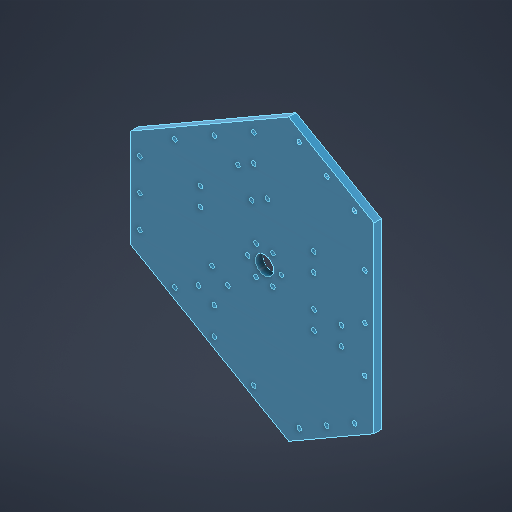
# Autodesk Inventor part: đế trên
Saved by Autodesk Inventor 2027.1 (Build 311270010, 270A)
## iProperties
Created: 2026-08-08
Part Number: đế trên
Material: Generic
Document SubType Name: Sheet Metal
Designer: MSI
Density: 1 g/cm^3
Sheet Metal Rule: Default_mm
Appearance: Sky Blue Dark
Author: MSI
Autodesk Inventor part; units mm, degrees
ref_plane "YZ Plane" through (0, 0, 0) normal (1, 0, 0) x (0, 1, 0)
ref_plane "XZ Plane" through (0, 0, 0) normal (0, 1, 0) x (-1, 0, 0)
ref_plane "XY Plane" through (0, 0, 0) normal (0, 0, 1) x (1, 0, 0)
sketch "Sketch1" plane through (0, 0, 0) normal (0, 0, 1) x (1, 0, 0)
  line L0 (120, 0) -> (120, -100)
  line L1 (120, 0) -> (120, 100)
  line L2 (-60, 103.923) -> (26.6025, 153.923)
  line L3 (-60, 103.923) -> (-146.6025, 53.923)
  line L4 (-60, -103.923) -> (-146.6025, -53.923)
  line L5 (-60, -103.923) -> (26.6025, -153.923)
  line L6 (26.6025, 153.923) -> (120, 100)
  line L7 (120, -100) -> (26.6025, -153.923)
  line L8 (-146.6025, -53.923) -> (-146.6025, 53.923)
  circle A0 centre (0, 0) radius 10
  dimension "d5" = 360
  constraints: 18 end point, 3 vertical, 1 centre point, 1 coincident, 16 other
extrude "Extrusion1" add sketch "Sketch1" along normal blind 8
sketch "Sketch2" plane through (0, 0, 8) normal (0, 0, 1) x (1, 0, 0)
  circle A0 centre (84.2544, -15) radius 2.5
  line L0 (120, -100) -> (120, 100) projected
  circle A1 centre (84.2544, -35) radius 2.5
  circle A2 centre (54.2544, -15) radius 2.5
  circle A3 centre (54.2544, -35) radius 2.5
  circle A4 centre (-14.1368, 54.4857) radius 2.5
  circle A5 centre (-29.1368, 80.4664) radius 2.5
  circle A6 centre (-11.8163, 90.4664) radius 2.5
  circle A7 centre (3.1837, 64.4857) radius 2.5
  circle A8 centre (-40.1176, -39.4857) radius 2.5
  circle A9 centre (-55.1176, -65.4664) radius 2.5
  circle A10 centre (-72.4381, -55.4664) radius 2.5
  circle A11 centre (-57.4381, -29.4857) radius 2.5
  point P0 (0, 0)
  point P1 (120, 0)
  dimension "d11" = 5
  dimension "d12" = 15
  dimension "d13" = 5
  dimension "d14" = 20
  dimension "d15" = 5
  dimension "d16" = 5
  dimension "d17" = 20
  dimension "d18" = 30
  dimension "d21" = 360
  constraints: 12 centre point, 1 midpoint, 25 other
  measures "d11" diameter of A0
  measures "d12" vertical distance of point (120, 0) A0.centre
  measures "d13" diameter of A1
  measures "d14" distance of A1.centre A0.centre
  measures "d15" diameter of A2
  measures "d16" diameter of A3
  measures "d17" distance of A3.centre A2.centre
  measures "d18" distance of A1.centre A3.centre
extrude "Extrusion2" cut sketch "Sketch2" against normal blind 8
sketch "Sketch3" plane through (0, 0, 8) normal (0, 0, 1) x (1, 0, 0)
  circle A0 centre (-136.6025, 35) radius 2.5
  circle A1 centre (-136.6025, 0) radius 2.5
  circle A2 centre (-136.6025, -35) radius 2.5
  line L0 (-146.6025, 53.923) -> (-146.6025, -53.923) projected
  circle A3 centre (37.9904, -135.8013) radius 2.5
  circle A4 centre (68.3013, -118.3013) radius 2.5
  circle A5 centre (98.6122, -100.8013) radius 2.5
  circle A6 centre (98.6122, 100.8013) radius 2.5
  circle A7 centre (68.3013, 118.3013) radius 2.5
  circle A8 centre (37.9904, 135.8013) radius 2.5
  point P0 (0, 0)
  point P1 (-146.6025, 0)
  point P2 (-146.6025, 0)
  dimension "d25" = 5
  dimension "d26" = 5
  dimension "d27" = 5
  dimension "d28" = 35
  dimension "d29" = 35
  dimension "d30" = 0
  dimension "d33" = 360
  dimension "d82" = 10
  dimension "d83" = 10
  constraints: 9 centre point, 2 midpoint, 19 other
  measures "d25" diameter of A0
  measures "d26" diameter of A1
  measures "d27" diameter of A2
  measures "d28" distance of A1.centre A0.centre
  measures "d29" distance of A2.centre A1.centre
  measures "d30" vertical distance of point (-146.603, 0) A1.centre
  measures "d82" distance from line of L0 A0.centre
  measures "d83" distance of point (-146.603, 0) A1.centre
extrude "Extrusion3" cut sketch "Sketch3" against normal blind 8
sketch "Sketch5" plane through (0, 0, 8) normal (0, 0, 1) x (1, 0, 0)
  circle A0 centre (18.3712, 0) radius 2.5
  circle A1 centre (9.1856, 15.9099) radius 2.5
  circle A2 centre (-9.1856, 15.9099) radius 2.5
  circle A3 centre (-18.3712, 0) radius 2.5
  circle A4 centre (-9.1856, -15.9099) radius 2.5
  circle A5 centre (9.1856, -15.9099) radius 2.5
  point P0 (0, 0)
  dimension "d51" = 5
  dimension "d54" = 360
  constraints: 6 centre point, 13 other
  measures "d51" diameter of A0
extrude "Extrusion5" cut sketch "Sketch5" against normal blind 8
sketch "Sketch6" plane through (0, 0, 8) normal (0, 0, 1) x (1, 0, 0)
  circle A0 centre (53.9473, 40) radius 2.5
  circle A1 centre (53.9473, 20) radius 2.5
  line L0 (120, -100) -> (120, 100) projected
  circle A2 centre (-70.3891, 40) radius 2.5
  circle A3 centre (-70.3891, 20) radius 2.5
  point P0 (0, 0)
  point P1 (120, 0)
  dimension "d58" = 5
  dimension "d59" = 5
  dimension "d60" = 20
  dimension "d61" = 20
  dimension "d62" = 5
  dimension "d63" = 5
  dimension "d64" = 20
  constraints: 4 centre point, 1 midpoint
  measures "d58" diameter of A0
  measures "d59" diameter of A1
  measures "d60" vertical distance of point (120, 0) A1.centre
  measures "d61" distance of A1.centre A0.centre
  measures "d62" diameter of A2
  measures "d63" diameter of A3
  measures "d64" distance of A3.centre A2.centre
extrude "Extrusion6" cut sketch "Sketch6" against normal blind 8
sketch "Sketch7" plane through (0, 0, 8) normal (0, 0, 1) x (1, 0, 0)
  circle A0 centre (110, 0) radius 2.5
  circle A1 centre (110, 50) radius 2.5
  circle A2 centre (110, -50) radius 2.5
  line L0 (120, -100) -> (120, 100) projected
  circle A3 centre (-98.3013, 70.2628) radius 2.5
  circle A4 centre (-55, 95.2628) radius 2.5
  circle A5 centre (-11.6987, 120.2628) radius 2.5
  circle A6 centre (-11.6987, -120.2628) radius 2.5
  circle A7 centre (-55, -95.2628) radius 2.5
  circle A8 centre (-98.3013, -70.2628) radius 2.5
  point P0 (0, 0)
  point P1 (120, 0)
  point P2 (120, 0)
  point P3 (120, 0)
  dimension "d68" = 5
  dimension "d69" = 5
  dimension "d70" = 5
  dimension "d71" = 50
  dimension "d72" = 50
  dimension "d75" = 360
  dimension "d77" = 10
  dimension "d78" = 10
  dimension "d79" = 10
  constraints: 9 centre point, 3 midpoint, 19 other
  measures "d68" diameter of A0
  measures "d69" diameter of A1
  measures "d70" diameter of A2
  measures "d71" vertical distance of point (120, 0) A1.centre
  measures "d72" vertical distance of point (120, 0) A2.centre
  measures "d77" distance of point (120, 0) A0.centre
  measures "d78" distance from line of L0 A1.centre
  measures "d79" distance from line of L0 A2.centre
extrude "Extrusion7" cut sketch "Sketch7" against normal blind 8
equation "\"BendRadius\" = Thickness"
equation "\"BendReliefWidth\" = Thickness"
equation "\"BendReliefDepth\" = 0.5 * Thickness"
equation "\"CornerReliefSize\" = 4 * Thickness"
equation "\"MinimumRemnant\" = 2 * Thickness"
equation "\"TransitionRadius\" = BendRadius"
equation "\"JacobiRadiusSize\" = BendRadius"
equation "\"GapSize\" = Thickness"
equation "\"Thickness\" = 0.5"
body "Solid1"
